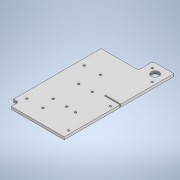
# Autodesk Inventor part: Inner Top Plate
Saved by Autodesk Inventor 2021 (Build 250183000, 183)
## iProperties
Created: 2020-07-16
Part Number: Inner Top Plate
Material: Generic
Document SubType Name: Modeling
Designer: jgray
Density: 1 g/cm^3
Appearance: Default
Author: jgray
Autodesk Inventor part; units mm, degrees
ref_plane "YZ Plane" through (0, 0, 0) normal (1, 0, 0) x (0, 1, 0)
ref_plane "XZ Plane" through (0, 0, 0) normal (0, 1, 0) x (-1, 0, 0)
ref_plane "XY Plane" through (0, 0, 0) normal (0, 0, 1) x (1, 0, 0)
sketch "Sketch1" plane through (0, 0, 0) normal (0, 1, 0) x (-1, 0, 0)
  line L0 (-55.6, 105) -> (55.6, 105)
  line L1 (55.6, 105) -> (55.6, -105)
  line L2 (55.6, -105) -> (-55.6, -105)
  line L3 (-55.6, -105) -> (-55.6, 105)
  line L4 (-55.6, 105) -> (55.6, -105) construction
  line L5 (55.6, 105) -> (-55.6, -105) construction
  line L6 (55.6, -105) -> (-15.6, -105)
  line L7 (-15.6, -105) -> (-15.6, -95)
  line L8 (-15.6, -95) -> (55.6, -95)
  line L9 (55.6, -95) -> (55.6, -105)
  line L10 (55.6, 105) -> (45.6, 105)
  line L11 (45.6, 105) -> (45.6, 95)
  line L12 (49.6, 91) -> (55.6, 91)
  line L13 (55.6, 91) -> (55.6, 105)
  arc A0 (45.6, 95) -> (49.6, 91) centre (49.6, 95) ccw
  point P0 (0, 0)
  point P1 (-15.6, -105)
  point P2 (55.6, -95)
  point P3 (55.6, 91)
  dimension "d0" = 111.2
  dimension "d1" = 210
  dimension "d84" = 10
  dimension "d85" = 40
  dimension "d86" = 14
  dimension "d87" = 10
  dimension "d88" = 4
  constraints: 28 end point, 6 parallel, 3 horizontal, 3 perpendicular, 2 midpoint, 2 point on circle, 2 tangent, 1 centre point
  measures "d0" distance of L1.end L2.end
  measures "d1" distance of L0.end L1.end
  measures "d84" distance of L6.end L7.end
  measures "d85" distance between parallel lines of L3 L7
  measures "d86" distance between parallel lines of L0 L12
  measures "d87" distance between parallel lines of L1 L11
  measures "d88" radius of A0
extrude "Extrusion1" add sketch "Sketch1" along normal blind 5 contours L0 L11 A0 L12 L1 L8 L7 L2 L3
sketch "Sketch2" plane through (0, 5, 0) normal (0, 1, 0) x (1, 0, 0)
  line L0 (36, 32.5) -> (-43.6, 32.5) construction
  line L1 (-43.6, -77.5) -> (36, -77.5) construction
  line L2 (-55.6, 95) -> (-55.6, -91) construction
  line L3 (-45.6, -105) -> (55.6, -105) projected
  point P0 (0, 0)
  point P1 (-12.6, -77.5)
  point P2 (-12.6, 32.5)
  dimension "d6" = 31
  dimension "d7" = 31
  dimension "d17" = 12
  dimension "d18" = 12
  dimension "d89" = 110
  dimension "d90" = 27.5
  constraints: 4 end point, 2 coincident, 2 point on line, 1 horizontal, 1 parallel
  measures "d6" distance of point (-12.6, -77.5) point (-43.6, -77.5)
  measures "d7" distance of point (-43.6, 32.5) point (-12.6, 32.5)
  measures "d17" distance from line of point (-43.6, 32.5) L2
  measures "d18" distance from line of point (-43.6, -77.5) L2
  measures "d89" distance between parallel lines of L1 L0
  measures "d90" distance between parallel lines of L1 L3
hole "Hole1" at (-43.6, 5, 77.5) at (-43.6, 5, -32.5) at (-12.6, 5, 77.5) at (-12.6, 5, -32.5) direction (0, -1, 0) diameter 3.8 end through all
sketch "Sketch6" plane through (0, 5, 0) normal (0, 1, 0) x (1, 0, 0)
  line L0 (25.9, 93.5) -> (-42.1, 93.5)
  line L1 (-42.1, 93.5) -> (-42.1, -53.5)
  line L2 (-42.1, -53.5) -> (25.9, -53.5)
  line L3 (25.9, -53.5) -> (25.9, 93.5)
  line L4 (25.9, 93.5) -> (-42.1, -53.5) construction
  line L5 (-42.1, 93.5) -> (25.9, -53.5) construction
  line L6 (55.6, -105) -> (55.6, 105) projected
  line L7 (-45.6, -105) -> (55.6, -105) projected
  line L8 (55.6, 105) -> (15.6, 105) projected
  point P0 (0, 0)
  point P1 (-8.1, 20)
  dimension "d29" = 68
  dimension "d30" = 147
  dimension "d32" = 29.7
  dimension "d91" = 51.5
  dimension "d92" = 11.5
  constraints: 12 end point, 4 coincident, 2 midpoint, 2 parallel, 1 horizontal, 1 perpendicular
  measures "d29" distance of L2.end L1.end
  measures "d30" distance of L1.end L0.end
  measures "d32" distance between parallel lines of L6 L3
  measures "d91" distance between parallel lines of L7 L2
  measures "d92" distance from line of L8 point (25.9, 93.5)
hole "Hole2" at (25.9, 5, -93.5) at (25.9, 5, 53.5) direction (0, -1, 0) diameter 3.8 end through all
sketch "Sketch14" plane through (0, 5, 0) normal (0, 1, 0) x (1, 0, 0)
  line L0 (49.1, 119.5954) -> (49.1, -116.5639) construction
  line L1 (55.6, -105) -> (55.6, 105) construction
  line L2 (-45.6, -105) -> (55.6, -105) construction
  point P0 (0, 0)
  point P1 (49.1, 70)
  point P2 (49.1, -10)
  point P3 (49.1, -90)
  dimension "d93" = 6.5
  dimension "d94" = 15
  dimension "d95" = 80
  dimension "d96" = 80
  constraints: 3 point on line, 2 end point, 1 vertical
  measures "d93" distance between parallel lines of L1 L0
  measures "d94" distance from line of L2 point (49.1, -90)
  measures "d95" distance of point (49.1, -10) point (49.1, -90)
  measures "d96" distance of point (49.1, 70) point (49.1, -10)
hole "Hole5" at (49.1, 5, -70) at (49.1, 5, 10) at (49.1, 5, 90) direction (0, -1, 0) diameter 3.8 end through all
sketch "Sketch13" plane through (0, 5, 0) normal (0, 1, 0) x (1, 0, 0)
  line L0 (25.9, 3) -> (25.9, -107.0389) construction
  circle A0 centre (25.9, 93.5) radius 1.9 construction
  circle A1 centre (25.9, -53.5) radius 1.9 construction
  circle A2 centre (-12.6, -77.5) radius 1.9 construction
  circle A3 centre (-43.6, -77.5) radius 1.9 construction
  circle A4 centre (-43.6, 32.5) radius 1.9 construction
  circle A5 centre (-12.6, 32.5) radius 1.9 construction
  line L1 (-55.6, 95) -> (-55.6, -91) construction
  line L2 (55.6, 1.7) -> (26.4, 1.7)
  line L3 (25.9, 2.2) -> (25.9, 3.5)
  line L4 (26.4, 3.5) -> (55.6, 3.5)
  line L5 (55.6, 3.5) -> (55.6, 1.7)
  arc A6 (26.4, 3.5) -> (25.9, 3) centre (26.4, 3) ccw
  arc A7 (25.9, 2.2) -> (26.4, 1.7) centre (26.4, 2.2) ccw
  line L6 (55.6, 105) -> (15.6, 105) projected
  line L7 (15.6, 105) -> (15.6, 95) projected
  line L8 (15.6, 95) -> (-55.6, 95) projected
  line L9 (-55.6, -91) -> (-49.6, -91) projected
  arc A8 (-45.6, -95) -> (-49.6, -91) centre (-49.6, -95) ccw projected
  line L10 (-45.6, -95) -> (-45.6, -105) projected
  line L11 (-45.6, -105) -> (55.6, -105) projected
  line L12 (55.6, -105) -> (55.6, 105) projected
  point P0 (0, 0)
  point P1 (25.9, 3)
  dimension "d75" = 1.8
  dimension "d76" = 0.5
  dimension "d77" = 90
  dimension "d78" = 57
  constraints: 10 end point, 4 point on circle, 4 tangent, 3 point on line, 2 centre point, 2 parallel, 1 equal radius, 1 horizontal, 1 perpendicular, 1 vertical
  measures "d75" distance between parallel lines of L2 L4
  measures "d76" radius of A6
  measures "d77" distance from line of A0.centre L4
  measures "d78" distance from line of A1.centre L4
extrude "Extrusion9" cut sketch "Sketch13" against normal through all
sketch "Sketch15" plane through (0, 5, 0) normal (0, 1, 0) x (1, 0, 0)
  line L0 (-18.1, -3.5) -> (7.9, -3.5) construction
  line L1 (7.9, -3.5) -> (7.9, -52.5) construction
  line L2 (7.9, -52.5) -> (-18.1, -52.5) construction
  line L3 (-18.1, -52.5) -> (-18.1, -3.5) construction
  circle A0 centre (-12.6, -77.5) radius 1.9 construction
  circle A1 centre (25.9, -53.5) radius 1.9 construction
  point P0 (0, 0)
  dimension "d104" = 26
  dimension "d105" = 49
  dimension "d106" = 25
  dimension "d107" = 18
  constraints: 8 end point, 4 coincident, 2 parallel, 1 horizontal, 1 perpendicular
  measures "d104" distance of L1.end L2.end
  measures "d105" distance of L0.end L1.end
  measures "d106" distance from line of L2 A0.centre
  measures "d107" horizontal distance of point (7.9, -52.5) A1.centre
hole "Hole6" at (-18.1, 5, 3.5) at (7.9, 5, 3.5) at (7.9, 5, 52.5) at (-18.1, 5, 52.5) direction (0, -1, 0) diameter 3.8 end through all
sketch "Sketch16" plane through (0, 5, 0) normal (0, 1, 0) x (1, 0, 0)
  line L0 (-55.6, 95) -> (-55.6, -91) projected
  line L1 (-55.6, 95) -> (15.6, 95)
  line L2 (15.6, 95) -> (15.6, 77)
  line L3 (15.6, 77) -> (-55.6, 77)
  line L4 (-55.6, 77) -> (-55.6, 95)
  line L5 (15.6, 105) -> (15.6, 95) projected
  circle A0 centre (38.5, 86.3) radius 7.5
  line L6 (55.6, 105) -> (15.6, 105) projected
  line L7 (55.6, 3.5) -> (55.6, 105) projected
  point P0 (0, 0)
  dimension "d115" = 18
  dimension "d116" = 15
  dimension "d117" = 18.7
  dimension "d118" = 17.1
  constraints: 8 end point, 2 parallel, 1 centre point, 1 collinear, 1 horizontal, 1 perpendicular
  measures "d115" distance between parallel lines of L1 L3
  measures "d116" diameter of A0
  measures "d117" distance from line of L6 A0.centre
  measures "d118" distance from line of L7 A0.centre
extrude "Extrusion10" cut sketch "Sketch16" against normal through all
fillet "Fillet1" radius 4 2 edges at (15.6, 2.5, -77) (15.6, 2.5, -105)
body "Solid1"
